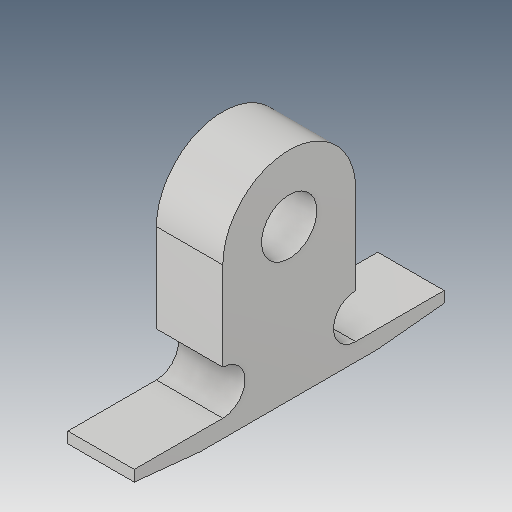
# Autodesk Inventor part: tip2
Saved by Autodesk Inventor 2019.4 (Build 234330000, 330)
## iProperties
Created: 2019-06-11
Part Number: tip2
Material: アルミニウム 2014-T4
Document SubType Name: Modeling
Designer: AzLIer
Density: 2.8 g/cm^3
Appearance: サテン
Mass: 0.440049 g
Surface Area: 2.68549 cm^2
Volume: 0.157161 cm^3
Author: AzLIer
Autodesk Inventor part; units mm, degrees
ref_plane "YZ Plane" through (0, 0, 0) normal (1, 0, 0) x (0, 1, 0)
ref_plane "XZ Plane" through (0, 0, 0) normal (0, 1, 0) x (-1, 0, 0)
ref_plane "XY Plane" through (0, 0, 0) normal (0, 0, 1) x (1, 0, 0)
sketch "スケッチ1" plane through (0, 0, 0) normal (1, 0, 0) x (0, 1, 0)
  line L0 (9, 0) -> (-9, 0) construction
  line L1 (9, 3) -> (-9, 3)
  line L2 (-9, -3) -> (9, -3)
  arc A0 (9, -3) -> (9, 3) centre (9, 0) ccw
  arc A1 (-9, 3) -> (-9, -3) centre (-9, 0) ccw
  line L3 (3, 7) -> (-3, 7)
  line L4 (-3, -7) -> (3, -7)
  line L5 (3, 7) -> (-3, -7) construction
  line L6 (-3, 7) -> (3, -7) construction
  line L7 (-3, 7) -> (-3, 5)
  line L8 (3, 5) -> (3, 7)
  line L9 (3, -7) -> (3, -5)
  line L10 (3, -3) -> (3, 3)
  line L11 (-3, 3) -> (-3, -3)
  line L12 (-3, -5) -> (-3, -7)
  circle A2 centre (-9, 0) radius 1.25
  circle A3 centre (9, 0) radius 1.25
  line L13 (3, -5) -> (3, -3)
  line L14 (3, 3) -> (3, 5)
  line L15 (-3, 5) -> (-3, 3)
  line L16 (-3, -3) -> (-3, -5)
  point P0 (0, 0)
  dimension "d0" = 6
  dimension "d1" = 6
  dimension "d3" = 14
  dimension "d4" = 18
  dimension "d7" = 0
  dimension "d8" = 6
  dimension "d9" = 4
  dimension "d11" = 2.5
  dimension "d12" = 2.5
  constraints: 36 end point, 12 parallel, 4 centre point, 4 collinear, 4 point on circle, 4 tangent, 3 midpoint, 3 perpendicular, 2 coincident, 2 horizontal, 2 point on line
  measures "d0" diameter of A1
  measures "d1" distance of L4.start L4.end
  measures "d3" distance between parallel lines of L4 L3
  measures "d4" distance of L0.start L0.end
  measures "d7" distance between parallel lines of L8 L10
  measures "d8" distance between parallel lines of L8 L11
  measures "d9" distance from line of L10.start L4
  measures "d11" diameter of A2
  measures "d12" diameter of A3
extrude "押し出し1" add sketch "スケッチ1" along normal blind 3 contours A0 L2 L10 L1 | L10 L2 L11 L1 | L1 L15 L7 L3 L8 L14 | L11 L2 A1 L1 | L13 L9 L4 L12 L16 L2 | A2 | A3
sketch "スケッチ2" plane through (0, 0, 0) normal (-1, 0, 0) x (0, 0, 1)
  spline S0 degree 3 poles (-3.8743, -1.25) (-3.891, -1.25) (-3.9108, -1.2467) (-3.9405, -1.236) (-3.956, -1.2272) (-3.9769, -1.209) (-3.9865, -1.1969) (-3.9969, -1.1748) (-4, -1.1615) (-4, -1.15) knots -0.016775 -0.016775 -0.016775 -0.016775 -0.011755 -0.011755 -0.007303 -0.007303 -0.003437 -0.003437 0 0 0 0
  line L0 (-4, -1.15) -> (-4, 1.15)
  spline S1 degree 3 poles (-4, 1.15) (-4, 1.1615) (-3.9969, 1.1748) (-3.9865, 1.1969) (-3.9769, 1.209) (-3.956, 1.2272) (-3.9405, 1.236) (-3.9108, 1.2467) (-3.891, 1.25) (-3.8743, 1.25) knots 0 0 0 0 0.003437 0.003437 0.007303 0.007303 0.011755 0.011755 0.016775 0.016775 0.016775 0.016775
  line L1 (-3.8743, 1.25) -> (-3.1638, 1.25)
  line L2 (-3.1638, 1.25) -> (-3.1638, 0.47)
  spline S2 degree 3 poles (-3.1638, 0.47) (-3.2063, 0.4464) (-3.2462, 0.4188) (-3.3386, 0.3411) (-3.3965, 0.2704) (-3.4581, 0.1426) (-3.4766, 0.0658) (-3.4766, 0) (-3.4766, -0.0658) (-3.4581, -0.1426) (-3.3965, -0.2704) (-3.3386, -0.3411) (-3.2462, -0.4188) (-3.2063, -0.4464) (-3.1638, -0.47) knots -0.055942 -0.055942 -0.055942 -0.055942 -0.042582 -0.042582 -0.019736 -0.019736 0 0 0 0.019736 0.019736 0.042582 0.042582 0.055942 0.055942 0.055942 0.055942
  line L3 (-3.1638, -0.47) -> (-3.1638, -1.25)
  line L4 (-3.1638, -1.25) -> (-3.8743, -1.25)
  spline S3 degree 3 poles (4, -1.15) (4, -1.1615) (3.9969, -1.1748) (3.9865, -1.1969) (3.9769, -1.209) (3.956, -1.2272) (3.9405, -1.236) (3.9108, -1.2467) (3.891, -1.25) (3.8743, -1.25) knots 0 0 0 0 0.003437 0.003437 0.007303 0.007303 0.011755 0.011755 0.016775 0.016775 0.016775 0.016775
  line L5 (3.8743, -1.25) -> (3.1638, -1.25)
  line L6 (3.1638, -1.25) -> (3.1638, -0.47)
  spline S4 degree 3 poles (3.1638, -0.47) (3.2063, -0.4464) (3.2462, -0.4188) (3.3386, -0.3411) (3.3965, -0.2704) (3.4581, -0.1426) (3.4766, -0.0658) (3.4766, 0) (3.4766, 0.0658) (3.4581, 0.1426) (3.3965, 0.2704) (3.3386, 0.3411) (3.2462, 0.4188) (3.2063, 0.4464) (3.1638, 0.47) knots -0.055942 -0.055942 -0.055942 -0.055942 -0.042582 -0.042582 -0.019736 -0.019736 0 0 0 0.019736 0.019736 0.042582 0.042582 0.055942 0.055942 0.055942 0.055942
  line L7 (3.1638, 0.47) -> (3.1638, 1.25)
  line L8 (3.1638, 1.25) -> (3.8743, 1.25)
  spline S5 degree 3 poles (3.8743, 1.25) (3.891, 1.25) (3.9108, 1.2467) (3.9405, 1.236) (3.956, 1.2272) (3.9769, 1.209) (3.9865, 1.1969) (3.9969, 1.1748) (4, 1.1615) (4, 1.15) knots -0.016775 -0.016775 -0.016775 -0.016775 -0.011755 -0.011755 -0.007303 -0.007303 -0.003437 -0.003437 0 0 0 0
  line L9 (4, 1.15) -> (4, -1.15)
  circle A0 centre (0, 9) radius 1.25 projected
  circle A1 centre (0, -9) radius 1.25 projected
  line L10 (-3, 3) -> (-7, 3) projected
  line L11 (-7, 3) -> (-7, -3) projected
  line L12 (-7, -3) -> (-3, -3) projected
  line L13 (-3, -3) -> (-3, -9) projected
  arc A2 (-3, -9) -> (3, -9) centre (0, -9) ccw projected
  line L14 (3, -9) -> (3, -3) projected
  line L15 (3, -3) -> (7, -3) projected
  line L16 (7, -3) -> (7, 3) projected
  line L17 (7, 3) -> (3, 3) projected
  line L18 (3, 3) -> (3, 9) projected
  arc A3 (3, 9) -> (-3, 9) centre (0, 9) ccw projected
  line L19 (-3, 9) -> (-3, 3) projected
  line L20 (-7, 2.5) -> (-4, 2.2)
  line L21 (-4, 2.2) -> (4, 2.2)
  line L22 (4, 2.2) -> (7, 2.5)
  arc A4 (-3, 3) -> (-3, 5) centre (-3, 4) ccw
  arc A5 (3, 5) -> (3, 3) centre (3, 4) ccw
  line L23 (3, 3) -> (3, 9) projected
  line L24 (-3, 9) -> (-3, 3) projected
  point P0 (0, 0)
  point P1 (0, 2.2)
  dimension "d15" = 2
  dimension "d17" = 8
  dimension "d18" = 0.8
  dimension "d19" = 0.5
  constraints: 28 end point, 7 point on line, 6 vertical, 5 horizontal, 4 point on circle, 2 centre point, 2 coincident, 1 equal length, 1 equal radius, 1 horizontal alignment, 1 midpoint, 1 vertical alignment, 28 other
  measures "d15" diameter of A4
  measures "d17" distance of L20.end L21.end
  measures "d18" distance between parallel lines of L10 L21
  measures "d19" distance from line of L10 L20.start
extrude "押し出し4" cut sketch "スケッチ2" against normal through all contours A4 L19 A3 L18 A5 L17 L16 L22 L21 L20 L11 L10 keep common part
